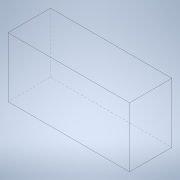
# Autodesk Inventor part: WaterCube
Saved by Autodesk Inventor 2022 (Build 260153000, 153)
## iProperties
Created: 2021-07-08
Part Number: WaterCube
Material: Generic
Document SubType Name: Modeling
Designer: jamieson-bl
Density: 1 g/cm^3
Appearance: Default
Author: jamieson-bl
Autodesk Inventor part; units mm, degrees
ref_plane "YZ Plane" through (0, 0, 0) normal (1, 0, 0) x (0, 1, 0)
ref_plane "XZ Plane" through (0, 0, 0) normal (0, 1, 0) x (-1, 0, 0)
ref_plane "XY Plane" through (0, 0, 0) normal (0, 0, 1) x (1, 0, 0)
sketch "Sketch1" plane through (0, 0, 0) normal (0, 0, 1) x (1, 0, 0)
  line L0 (1200.15, -590.55) -> (-1200.15, -590.55)
  line L1 (-1200.15, -590.55) -> (-1200.15, 590.55)
  line L2 (-1200.15, 590.55) -> (1200.15, 590.55)
  line L3 (1200.15, 590.55) -> (1200.15, -590.55)
  line L4 (1200.15, -590.55) -> (-1200.15, 590.55) construction
  line L5 (-1200.15, -590.55) -> (1200.15, 590.55) construction
  point P0 (0, 0)
  dimension "d0" = 2400.3
  dimension "d1" = 1181.1
  constraints: 12 end point, 2 midpoint, 2 parallel, 1 horizontal, 1 perpendicular
  measures "d0" distance of L1.end L2.end
  measures "d1" distance of L0.end L1.end
extrude "Extrusion1" add sketch "Sketch1" along normal blind 838.2
